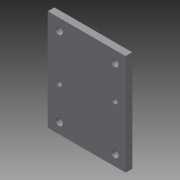
# Autodesk Inventor part: m
Saved by Autodesk Inventor 2015 (Build 190159000, 159)
## iProperties
Created: 2015-11-06
Part Number: m
Material: Generic
Document SubType Name: Modeling
Designer: EriveltonDell
Density: 1 g/cm^3
Appearance: Default
Author: EriveltonDell
Autodesk Inventor part; units mm, degrees
ref_plane "YZ Plane" through (0, 0, 0) normal (1, 0, 0) x (0, 1, 0)
ref_plane "XZ Plane" through (0, 0, 0) normal (0, 1, 0) x (-1, 0, 0)
ref_plane "XY Plane" through (0, 0, 0) normal (0, 0, 1) x (1, 0, 0)
sketch "Sketch1" plane through (0, 0, 0) normal (0, 1, 0) x (-1, 0, 0)
  line L0 (-14, -58.75) -> (-19, -58.75)
  line L1 (-35.25, 21.625) -> (35.25, 21.625)
  line L2 (-35.25, 21.625) -> (35.25, 21.625) construction
  line L3 (35.25, 21.625) -> (25.25, 21.625)
  line L4 (-35.25, 21.625) -> (35.25, 21.625)
  line L5 (35.25, 21.625) -> (35.25, -69.875)
  line L6 (35.25, -69.875) -> (-35.25, -69.875)
  line L7 (-35.25, -69.875) -> (-35.25, 21.625)
  line L8 (-35.25, 21.625) -> (-35.25, 11.625)
  line L9 (-35.25, 11.625) -> (-25.25, 11.625)
  circle A0 centre (-25.25, 11.625) radius 3.5
  line L10 (35.25, 21.625) -> (25.25, 21.625)
  line L11 (25.25, 21.625) -> (25.25, 11.625)
  circle A1 centre (25.25, 11.625) radius 3.5
  line L12 (35.25, -69.875) -> (25.25, -69.875)
  line L13 (25.25, -69.875) -> (25.25, -59.875)
  circle A2 centre (25.25, -59.875) radius 3.5
  line L14 (-35.25, -69.875) -> (-25.25, -69.875)
  line L15 (-25.25, -69.875) -> (-25.25, -59.875)
  circle A3 centre (-25.25, -59.875) radius 3.5
  line L16 (-25.25, 11.625) -> (-25.25, -18.375)
  line L17 (25.25, -59.875) -> (25.25, -29.875)
  circle A4 centre (-25.25, -18.375) radius 2.5
  circle A5 centre (25.25, -29.875) radius 2.5
  point P0 (0, 0)
  dimension "d6" = 5
  dimension "d9" = 70.5
  dimension "d41" = 70.5
  dimension "d42" = 91.5
  dimension "d43" = 10
  dimension "d44" = 10
  dimension "d45" = 7
  dimension "d46" = 10
  dimension "d47" = 10
  dimension "d48" = 90
  dimension "d50" = 7
  dimension "d51" = 10
  dimension "d52" = 10
  dimension "d53" = 7
  dimension "d54" = 10
  dimension "d55" = 10
  dimension "d56" = 7
  dimension "d60" = 30
  dimension "d61" = 30
  dimension "d62" = 5
  dimension "d63" = 5
  constraints: 36 end point, 6 centre point, 6 coincident, 5 perpendicular, 4 point on line, 3 equal length, 3 horizontal, 2 vertical, 1 collinear
  measures "d6" distance of L0.start L0.end
  measures "d9" distance of L1.start L1.end
  measures "d41" distance of L5.end L6.end
  measures "d42" distance of L4.end L5.end
  measures "d43" distance of L1.start L8.end
  measures "d44" distance of L8.end L9.end
  measures "d45" diameter of A0
  measures "d46" distance of L4.end L3.end
  measures "d47" distance of L3.end L11.end
  measures "d48" angle of L11 L10
  measures "d50" diameter of A1
  measures "d51" distance of L5.end L12.end
  measures "d52" distance of L12.end L13.end
  measures "d53" diameter of A2
  measures "d54" distance of L6.end L14.end
  measures "d55" distance of L14.end L15.end
  measures "d56" diameter of A3
  measures "d60" distance of L16.start L16.end
  measures "d61" distance of L17.start L17.end
  measures "d62" diameter of A4
  measures "d63" diameter of A5
extrude "Extrusion1" add sketch "Sketch1" along normal blind 6
body "Solid1"
